Autodesk Fusion 360 part; units mm, degrees
note: some values were not read from the file. Chosen so that the rebuilt part matches the saved one: which bodies a step acts on; which face or edge a step refers to. Set by a fixed rule: which sketch regions a step uses.
(part 3 of 3)
sketch "Schizzo6 (2)" plane through (0, 86.5, 0) normal (0, -1, 0) x (1, 0, 0)
  line L0 (-43.5, 106) -> (-43.5, 111)
  line L1 (-43.5, 111) -> (-33.5, 111)
  line L2 (-33.5, 111) -> (-33.5, 176)
  line L3 (-33.5, 176) -> (-116.5, 176)
  line L4 (-116.5, 176) -> (-116.5, 111)
  line L5 (-116.5, 111) -> (-106.5, 111)
  line L6 (-106.5, 111) -> (-106.5, 106)
  line L7 (-106.5, 106) -> (-116.5, 106)
  line L8 (-116.5, 106) -> (-116.5, 101)
  line L9 (-116.5, 101) -> (-33.5, 101)
  line L10 (-33.5, 101) -> (-33.5, 106)
  line L11 (-33.5, 106) -> (-43.5, 106)
  line L12 (-116.5, 111) -> (-116.5, 128.3205)
  line L13 (-106.5, 111) -> (-116.5, 111)
  line L14 (-106.5, 111) -> (-116.5, 128.3205)
  line L15 (-106.5, 111) -> (-86.5, 111) construction
  dimension "d209" = 120
  constraint coincident L5.end L6.start
  constraint coincident L4 L12.end
  constraint coincident L4.end L5.start
  constraint perpendicular L5 L12
  constraint horizontal L15
  measures "d209" angle of L14 L15
revolve "Rivoluzione2" add sketch "Schizzo6 (2)" angle 90 about axis through (-116.5, 86.5, 176) along (0, 0, -1) contours L4 L5 L12 L13 L14 bodies 3 in component "Coperchio"
sketch "Schizzo7" plane through (0, 86.5, 0) normal (0, -1, 0) x (1, 0, 0)
  line L0 (-106.5, 111) -> (-106.5, 106)
  line L1 (-106.5, 106) -> (-116.5, 106)
  line L2 (-116.5, 106) -> (-116.5, 101)
  line L3 (-116.5, 101) -> (-33.5, 101)
  line L4 (-33.5, 101) -> (-33.5, 106)
  line L5 (-33.5, 106) -> (-43.5, 106)
  line L6 (-43.5, 106) -> (-43.5, 111)
  line L7 (-43.5, 111) -> (-33.5, 111)
  line L8 (-33.5, 111) -> (-33.5, 176)
  line L9 (-33.5, 176) -> (-116.5, 176)
  line L10 (-43.5, 111) -> (-33.5, 128.3287)
  line L11 (-33.5, 111) -> (-33.5, 128.3287)
  line L12 (-43.5, 111) -> (-33.5, 111)
  line L13 (-116.5, 128.3205) -> (-106.5, 111)
  line L14 (-116.5, 176) -> (-116.5, 128.3205)
  constraint coincident L6.end L7.start
  constraint coincident L8 L10.end
  constraint coincident L7.end L8.start
  constraint perpendicular L7 L11
revolve "Rivoluzione3" add sketch "Schizzo7" angle 90 about axis through (-33.5, 86.5, 111) along (0, 0, 1) contours L7 L8 L10 L11 L12 bodies 3 in component "Coperchio"
sketch "Schizzo8" plane through (0, 3.5, 0) normal (0, 1, 0) x (-1, 0, 0)
  line L0 (33.5, 102) -> (116.5, 102)
  line L1 (116.5, 102) -> (116.5, 106)
  line L2 (116.5, 106) -> (106.5, 106)
  line L3 (106.5, 106) -> (106.5, 111)
  line L4 (106.5, 111) -> (116.5, 111)
  line L5 (116.5, 111) -> (116.5, 176)
  line L6 (116.5, 176) -> (33.5, 176)
  line L7 (33.5, 176) -> (33.5, 111)
  line L8 (33.5, 111) -> (43.5, 111)
  line L9 (43.5, 111) -> (43.5, 106)
  line L10 (43.5, 106) -> (33.5, 106)
  line L11 (33.5, 106) -> (33.5, 102)
  line L12 (43.5, 111) -> (33.5, 128.3014)
  line L13 (33.5, 111) -> (43.5, 111)
  line L14 (33.5, 111) -> (33.5, 128.3014)
  constraint coincident L8.end L9.start
  constraint coincident L7 L12.end
  constraint coincident L7.end L8.start
  constraint perpendicular L8 L14
revolve "Rivoluzione4" add sketch "Schizzo8" angle 90 about axis through (-33.5, 3.5, 176) along (0, 0, -1) contours L7 L8 L12 L13 L14 bodies 3 in component "Coperchio"
sketch "Schizzo9 (2)" plane through (0, 3.5, 0) normal (0, 1, 0) x (-1, 0, 0)
  line L0 (33.5, 128.3014) -> (43.5, 111)
  line L1 (43.5, 111) -> (43.5, 106)
  line L2 (43.5, 106) -> (33.5, 106)
  line L3 (33.5, 106) -> (33.5, 102)
  line L4 (33.5, 102) -> (116.5, 102)
  line L5 (116.5, 102) -> (116.5, 106)
  line L6 (116.5, 106) -> (106.5, 106)
  line L7 (106.5, 106) -> (106.5, 111)
  line L8 (106.5, 111) -> (116.5, 111)
  line L9 (116.5, 111) -> (116.5, 176)
  line L10 (116.5, 176) -> (33.5, 176)
  line L11 (33.5, 176) -> (33.5, 128.3014)
  line L12 (116.5, 128.3205) -> (116.5, 111)
  line L13 (116.5, 111) -> (106.5, 111)
  line L14 (106.5, 111) -> (116.5, 128.3205)
  line L15 (106.5, 111) -> (126.5, 111) construction
  dimension "d210" = 60
  constraint coincident L7.end L8.start
  constraint coincident L9 L12.start
  constraint coincident L8.end L9.start
  constraint perpendicular L8 L12
  constraint horizontal L15
  measures "d210" angle of L14 L15
revolve "Rivoluzione5" add sketch "Schizzo9 (2)" angle 90 about axis through (-116.5, 3.5, 111) along (0, 0, 1) contours L8 L9 L12 L13 L14 bodies 3 in component "Coperchio"
fillet "Raccordo3'" radius 0.3 179 edges at (17.7456, 31.25, 16) (16.4456, 27.9642, 16) (19.0456, 27.9642, 16) (20.2223, 27.6, 16) (20.2223, 26.4, 16) (23.7456, 27, 16) (19.0456, 25.6, 16) (16.4456, 25.6, 16) (15.2688, 27.6, 16) (11.7456, 27, 16) (15.2688, 26.4, 16) (15.8206, 24.8, 16) (15.1956, 22.025, 16) (20.2956, 22.025, 16) (19.6706, 24.8, 16) (14.6438, 19.25, 16) (11.7456, 18.65, 16) (14.6438, 18.05, 16) (15.1956, 15.275, 16) (15.2688, 10.9, 16) (16.4456, 11.7, 16) (15.8206, 12.5, 16) (11.7456, 10.3, 16) (15.2688, 9.7, 16) (17.7456, 6.05, 16) (16.4456, 9.3358, 16) (19.0456, 9.3358, 16) (19.0456, 11.7, 16) (19.6706, 12.5, 16) (20.2223, 10.9, 16) (20.2223, 9.7, 16) (23.7456, 10.3, 16) (20.2956, 15.275, 16) (20.8473, 18.05, 16) (20.8473, 19.25, 16) (23.7456, 18.65, 16) (31.3706, 31.25, 16) (30.0706, 27.9642, 16) (28.8938, 27.6, 16) (25.3706, 27, 16) (28.8938, 26.4, 16) (32.6706, 27.9642, 16) (33.8473, 27.6, 16) (37.3706, 27, 16) (33.8473, 26.4, 16) (32.6706, 25.6, 16) (30.0706, 25.6, 16) (29.4456, 24.8, 16) (28.8206, 22.025, 16) (33.2956, 24.8, 16) (33.9206, 22.025, 16) (28.2688, 19.25, 16) (25.3706, 18.65, 16) (28.2688, 18.05, 16) (28.8206, 15.275, 16) (34.4723, 19.25, 16) (37.3706, 18.65, 16) (34.4723, 18.05, 16) (33.9206, 15.275, 16) (29.4456, 12.5, 16) (30.0706, 11.7, 16) (28.8938, 10.9, 16) (25.3706, 10.3, 16) (28.8938, 9.7, 16) (30.0706, 9.3358, 16) (31.3706, 6.05, 16) (32.6706, 9.3358, 16) (33.8473, 9.7, 16) (33.8473, 10.9, 16) (32.6706, 11.7, 16) (33.2956, 12.5, 16) (37.3706, 10.3, 16) (38.9956, 27, 16) (42.5188, 27.6, 16) (42.5188, 26.4, 16) (43.6956, 25.6, 16) (43.0706, 24.8, 16) (42.4456, 22.025, 16) (38.9956, 18.65, 16) (41.8938, 19.25, 16) (41.8938, 18.05, 16) (42.4456, 15.275, 16) (43.0706, 12.5, 16) (43.6956, 11.7, 16) (42.5188, 10.9, 16) (38.9956, 10.3, 16) (42.5188, 9.7, 16) (43.6956, 9.3358, 16) (44.9956, 6.05, 16) (47.4723, 9.7, 16) (46.2956, 11.7, 16) (46.2956, 9.3358, 16) (47.4723, 10.9, 16) (50.9956, 10.3, 16) (46.9206, 12.5, 16) (47.5456, 15.275, 16) (48.0973, 19.25, 16) (48.0973, 18.05, 16) (50.9956, 18.65, 16) (47.5456, 22.025, 16) (50.9956, 27, 16) (47.4723, 27.6, 16) (47.4723, 26.4, 16) (46.2956, 25.6, 16) (43.6956, 27.9642, 16) (44.9956, 31.25, 16) (46.2956, 27.9642, 16) (58.6206, 31.25, 16) (57.3206, 27.9642, 16) (59.9206, 27.9642, 16) (61.0973, 27.6, 16) (61.0973, 26.4, 16) (64.6206, 27, 16) (56.1438, 27.6, 16) (52.6206, 27, 16) (56.1438, 26.4, 16) (56.6956, 24.8, 16) (57.3206, 25.6, 16) (56.0706, 22.025, 16) (59.9206, 25.6, 16) (60.5456, 24.8, 16) (61.1706, 22.025, 16) (61.7223, 19.25, 16) (61.7223, 18.05, 16) (64.6206, 18.65, 16) (52.6206, 18.65, 16) (55.5188, 19.25, 16) (55.5188, 18.05, 16) (56.0706, 15.275, 16) (56.6956, 12.5, 16) (57.3206, 11.7, 16) (59.9206, 11.7, 16) (60.5456, 12.5, 16) (61.1706, 15.275, 16) (56.1438, 10.9, 16) (52.6206, 10.3, 16) (56.1438, 9.7, 16) (57.3206, 9.3358, 16) (58.6206, 6.05, 16) (59.9206, 9.3358, 16) (61.0973, 9.7, 16) (61.0973, 10.9, 16) (64.6206, 10.3, 16) (66.2456, 27, 16) (69.7688, 27.6, 16) (72.2456, 31.25, 16) (70.9456, 27.9642, 16) (73.5456, 27.9642, 16) (74.7223, 27.6, 16) (78.2456, 27, 16) (74.7223, 26.4, 16) (73.5456, 25.6, 16) (69.7688, 26.4, 16) (70.9456, 25.6, 16) (70.3206, 24.8, 16) (69.6956, 22.025, 16) (74.1706, 24.8, 16) (74.7956, 22.025, 16) (75.3473, 19.25, 16) (75.3473, 18.05, 16) (78.2456, 18.65, 16) (74.7956, 15.275, 16) (66.2456, 18.65, 16) (69.1438, 19.25, 16) (69.1438, 18.05, 16) (69.6956, 15.275, 16) (70.3206, 12.5, 16) (70.9456, 11.7, 16) (69.7688, 10.9, 16) (66.2456, 10.3, 16) (69.7688, 9.7, 16) (70.9456, 9.3358, 16) (72.2456, 6.05, 16) (73.5456, 9.3358, 16) (74.7223, 9.7, 16) (73.5456, 11.7, 16) (74.1706, 12.5, 16) (74.7223, 10.9, 16) (78.2456, 10.3, 16) on bodies 2 in component "Cubo"
fillet "Raccordo4'" radius 0.3 180 edges at (15.1956, 48.375, 16) (15.8206, 51.15, 16) (16.4456, 51.95, 16) (11.7456, 45, 16) (14.6438, 45.6, 16) (14.6438, 44.4, 16) (15.1956, 41.625, 16) (11.7456, 36.65, 16) (15.2688, 37.25, 16) (15.8206, 38.85, 16) (16.4456, 38.05, 16) (15.2688, 36.05, 16) (16.4456, 35.6858, 16) (17.7456, 32.4, 16) (19.0456, 38.05, 16) (19.6706, 38.85, 16) (20.2956, 41.625, 16) (20.2223, 37.25, 16) (20.2223, 36.05, 16) (19.0456, 35.6858, 16) (23.7456, 36.65, 16) (20.2956, 48.375, 16) (20.8473, 45.6, 16) (23.7456, 45, 16) (20.8473, 44.4, 16) (15.2688, 53.95, 16) (11.7456, 53.35, 16) (15.2688, 52.75, 16) (16.4456, 54.3142, 16) (17.7456, 57.6, 16) (19.0456, 54.3142, 16) (20.2223, 53.95, 16) (20.2223, 52.75, 16) (19.0456, 51.95, 16) (23.7456, 53.35, 16) (19.6706, 51.15, 16) (28.8206, 48.375, 16) (28.2688, 45.6, 16) (25.3706, 45, 16) (28.2688, 44.4, 16) (28.8206, 41.625, 16) (29.4456, 38.85, 16) (30.0706, 38.05, 16) (28.8938, 37.25, 16) (25.3706, 36.65, 16) (28.8938, 36.05, 16) (31.3706, 32.4, 16) (30.0706, 35.6858, 16) (32.6706, 35.6858, 16) (33.8473, 36.05, 16) (32.6706, 38.05, 16) (33.2956, 38.85, 16) (33.8473, 37.25, 16) (37.3706, 36.65, 16) (33.9206, 41.625, 16) (34.4723, 45.6, 16) (33.9206, 48.375, 16) (34.4723, 44.4, 16) (37.3706, 45, 16) (31.3706, 57.6, 16) (30.0706, 54.3142, 16) (28.8938, 53.95, 16) (25.3706, 53.35, 16) (28.8938, 52.75, 16) (30.0706, 51.95, 16) (29.4456, 51.15, 16) (32.6706, 51.95, 16) (33.8473, 53.95, 16) (32.6706, 54.3142, 16) (37.3706, 53.35, 16) (33.8473, 52.75, 16) (33.2956, 51.15, 16) (38.9956, 53.35, 16) (42.5188, 53.95, 16) (44.9956, 57.6, 16) (43.6956, 54.3142, 16) (46.2956, 54.3142, 16) (47.4723, 53.95, 16) (50.9956, 53.35, 16) (47.4723, 52.75, 16) (46.2956, 51.95, 16) (46.9206, 51.15, 16) (43.6956, 51.95, 16) (42.5188, 52.75, 16) (43.0706, 51.15, 16) (42.4456, 48.375, 16) (38.9956, 45, 16) (41.8938, 45.6, 16) (41.8938, 44.4, 16) (42.4456, 41.625, 16) (43.0706, 38.85, 16) (38.9956, 36.65, 16) (42.5188, 37.25, 16) (43.6956, 38.05, 16) (46.2956, 38.05, 16) (46.9206, 38.85, 16) (47.4723, 37.25, 16) (42.5188, 36.05, 16) (43.6956, 35.6858, 16) (44.9956, 32.4, 16) (46.2956, 35.6858, 16) (47.4723, 36.05, 16) (50.9956, 36.65, 16) (47.5456, 41.625, 16) (47.5456, 48.375, 16) (48.0973, 45.6, 16) (48.0973, 44.4, 16) (50.9956, 45, 16) (57.3206, 54.3142, 16) (58.6206, 57.6, 16) (56.1438, 53.95, 16) (52.6206, 53.35, 16) (56.1438, 52.75, 16) (57.3206, 51.95, 16) (56.6956, 51.15, 16) (56.0706, 48.375, 16) (55.5188, 45.6, 16) (52.6206, 45, 16) (55.5188, 44.4, 16) (56.0706, 41.625, 16) (56.6956, 38.85, 16) (57.3206, 38.05, 16) (56.1438, 37.25, 16) (52.6206, 36.65, 16) (56.1438, 36.05, 16) (57.3206, 35.6858, 16) (58.6206, 32.4, 16) (59.9206, 35.6858, 16) (59.9206, 38.05, 16) (61.0973, 37.25, 16) (61.0973, 36.05, 16) (61.1706, 41.625, 16) (60.5456, 38.85, 16) (64.6206, 36.65, 16) (61.7223, 44.4, 16) (61.7223, 45.6, 16) (61.1706, 48.375, 16) (64.6206, 45, 16) (60.5456, 51.15, 16) (59.9206, 51.95, 16) (61.0973, 52.75, 16) (61.0973, 53.95, 16) (59.9206, 54.3142, 16) (64.6206, 53.35, 16) (69.1438, 45.6, 16) (66.2456, 45, 16) (69.6956, 48.375, 16) (69.7688, 52.75, 16) (69.7688, 53.95, 16) (66.2456, 53.35, 16) (72.2456, 57.6, 16) (70.9456, 54.3142, 16) (70.9456, 51.95, 16) (70.3206, 51.15, 16) (69.1438, 44.4, 16) (69.6956, 41.625, 16) (70.3206, 38.85, 16) (70.9456, 38.05, 16) (69.7688, 37.25, 16) (66.2456, 36.65, 16) (69.7688, 36.05, 16) (70.9456, 35.6858, 16) (72.2456, 32.4, 16) (73.5456, 35.6858, 16) (73.5456, 38.05, 16) (74.1706, 38.85, 16) (74.7223, 37.25, 16) (74.7223, 36.05, 16) (78.2456, 36.65, 16) (74.7956, 41.625, 16) (74.7223, 53.95, 16) (73.5456, 54.3142, 16) (73.5456, 51.95, 16) (74.7223, 52.75, 16) (78.2456, 53.35, 16) (74.1706, 51.15, 16) (74.7956, 48.375, 16) (75.3473, 45.6, 16) (75.3473, 44.4, 16) (78.2456, 45, 16) on bodies 2 in component "Cubo"
fillet "Raccordo5" radius 0.3 180 edges at (17.7456, 83.95, 16) (16.4456, 80.6642, 16) (15.2688, 80.3, 16) (11.7456, 79.7, 16) (15.2688, 79.1, 16) (16.4456, 78.3, 16) (15.8206, 77.5, 16) (15.1956, 74.725, 16) (20.2223, 80.3, 16) (19.0456, 80.6642, 16) (20.2223, 79.1, 16) (23.7456, 79.7, 16) (19.0456, 78.3, 16) (19.6706, 77.5, 16) (20.2956, 74.725, 16) (14.6438, 71.95, 16) (11.7456, 71.35, 16) (14.6438, 70.75, 16) (15.1956, 67.975, 16) (20.8473, 71.95, 16) (23.7456, 71.35, 16) (20.8473, 70.75, 16) (20.2956, 67.975, 16) (19.6706, 65.2, 16) (19.0456, 64.4, 16) (16.4456, 64.4, 16) (15.8206, 65.2, 16) (15.2688, 63.6, 16) (15.2688, 62.4, 16) (11.7456, 63, 16) (20.2223, 63.6, 16) (20.2223, 62.4, 16) (23.7456, 63, 16) (16.4456, 62.0358, 16) (17.7456, 58.75, 16) (19.0456, 62.0358, 16) (28.8206, 74.725, 16) (28.2688, 71.95, 16) (25.3706, 71.35, 16) (25.3706, 79.7, 16) (28.8938, 80.3, 16) (28.8938, 79.1, 16) (30.0706, 78.3, 16) (29.4456, 77.5, 16) (30.0706, 80.6642, 16) (31.3706, 83.95, 16) (32.6706, 80.6642, 16) (33.8473, 80.3, 16) (33.8473, 79.1, 16) (32.6706, 78.3, 16) (33.2956, 77.5, 16) (33.9206, 74.725, 16) (37.3706, 79.7, 16) (34.4723, 71.95, 16) (37.3706, 71.35, 16) (34.4723, 70.75, 16) (33.9206, 67.975, 16) (28.8206, 67.975, 16) (28.2688, 70.75, 16) (29.4456, 65.2, 16) (30.0706, 64.4, 16) (28.8938, 63.6, 16) (33.2956, 65.2, 16) (32.6706, 64.4, 16) (33.8473, 63.6, 16) (37.3706, 63, 16) (33.8473, 62.4, 16) (30.0706, 62.0358, 16) (32.6706, 62.0358, 16) (31.3706, 58.75, 16) (28.8938, 62.4, 16) (25.3706, 63, 16) (42.5188, 80.3, 16) (43.6956, 80.6642, 16) (44.9956, 83.95, 16) (47.4723, 80.3, 16) (46.2956, 80.6642, 16) (50.9956, 79.7, 16) (47.4723, 79.1, 16) (46.2956, 78.3, 16) (46.9206, 77.5, 16) (47.5456, 74.725, 16) (42.5188, 79.1, 16) (43.6956, 78.3, 16) (43.0706, 77.5, 16) (42.4456, 74.725, 16) (38.9956, 79.7, 16) (41.8938, 71.95, 16) (41.8938, 70.75, 16) (38.9956, 71.35, 16) (42.4456, 67.975, 16) (38.9956, 63, 16) (42.5188, 63.6, 16) (42.5188, 62.4, 16) (43.6956, 64.4, 16) (43.0706, 65.2, 16) (46.9206, 65.2, 16) (47.5456, 67.975, 16) (48.0973, 70.75, 16) (48.0973, 71.95, 16) (50.9956, 71.35, 16) (46.2956, 64.4, 16) (47.4723, 63.6, 16) (47.4723, 62.4, 16) (46.2956, 62.0358, 16) (43.6956, 62.0358, 16) (44.9956, 58.75, 16) (50.9956, 63, 16) (55.5188, 71.95, 16) (56.0706, 74.725, 16) (55.5188, 70.75, 16) (56.0706, 67.975, 16) (56.6956, 65.2, 16) (57.3206, 64.4, 16) (56.1438, 63.6, 16) (52.6206, 63, 16) (56.1438, 62.4, 16) (57.3206, 62.0358, 16) (58.6206, 58.75, 16) (59.9206, 62.0358, 16) (61.0973, 62.4, 16) (61.0973, 63.6, 16) (59.9206, 64.4, 16) (60.5456, 65.2, 16) (61.1706, 67.975, 16) (64.6206, 63, 16) (61.1706, 74.725, 16) (60.5456, 77.5, 16) (56.1438, 79.1, 16) (57.3206, 78.3, 16) (56.6956, 77.5, 16) (61.7223, 71.95, 16) (61.7223, 70.75, 16) (64.6206, 71.35, 16) (61.0973, 79.1, 16) (61.0973, 80.3, 16) (59.9206, 80.6642, 16) (58.6206, 83.95, 16) (57.3206, 80.6642, 16) (56.1438, 80.3, 16) (52.6206, 79.7, 16) (59.9206, 78.3, 16) (64.6206, 79.7, 16) (52.6206, 71.35, 16) (72.2456, 83.95, 16) (70.9456, 80.6642, 16) (69.7688, 80.3, 16) (66.2456, 79.7, 16) (69.7688, 79.1, 16) (70.9456, 78.3, 16) (70.3206, 77.5, 16) (69.6956, 74.725, 16) (69.1438, 71.95, 16) (66.2456, 71.35, 16) (69.1438, 70.75, 16) (69.6956, 67.975, 16) (73.5456, 80.6642, 16) (74.7223, 80.3, 16) (78.2456, 79.7, 16) (74.7223, 79.1, 16) (73.5456, 78.3, 16) (74.1706, 77.5, 16) (74.7956, 74.725, 16) (75.3473, 71.95, 16) (78.2456, 71.35, 16) (75.3473, 70.75, 16) (74.7956, 67.975, 16) (74.1706, 65.2, 16) (73.5456, 64.4, 16) (70.3206, 65.2, 16) (70.9456, 64.4, 16) (69.7688, 63.6, 16) (66.2456, 63, 16) (69.7688, 62.4, 16) (70.9456, 62.0358, 16) (72.2456, 58.75, 16) (73.5456, 62.0358, 16) (74.7223, 62.4, 16) (74.7223, 63.6, 16) (78.2456, 63, 16) on bodies 2 in component "Cubo"
component "Cubo" placed x (1, 0, 0) y (0, 1, 0) z (0, 0, 1) at (0, 0, 0)
component "Coperchio" placed x (1, 0, 0) y (0, 1, 0) z (0, 0, 1) at (0, 0, 0) in component "Cubo"
hidden bodies 2
named bodies: "Coperchio", "Base"
